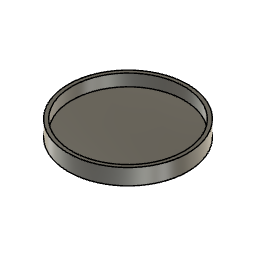
Piston Hood 1 (Autodesk Fusion 360 design; units mm, degrees)
Autodesk Fusion 360 part; units mm, degrees
sketch "Sketch1" plane through (0, 0, 0) normal (0, 0, 1) x (1, 0, 0) in component "Component"
  line L0 (3.8891, 2.4749) -> (5.2486, 3.8344)
  circle A0 centre (0, 0) radius 6.5
  line L1 (-2.4749, 3.8891) -> (-3.8344, 5.2486)
  circle A1 centre (0, 0) radius 7.05
  line L2 (3.182, 3.182) -> (2.4749, 3.8891)
  line L3 (-3.182, 3.182) -> (-3.8891, 2.4749)
  line L4 (-3.182, -3.182) -> (-2.4749, -3.8891)
  line L5 (-3.8891, -2.4749) -> (-5.2486, -3.8344)
  line L6 (2.4749, -3.8891) -> (3.8344, -5.2486)
  line L7 (-2.4749, -3.8891) -> (-3.8344, -5.2486)
  line L8 (3.182, -3.182) -> (2.4749, -3.8891)
  line L9 (-3.182, -3.182) -> (-3.8891, -2.4749)
  circle A2 centre (0, 0) radius 7.5
  line L10 (3.182, 3.182) -> (3.8891, 2.4749)
  line L11 (-3.8891, 2.4749) -> (-5.2486, 3.8344)
  line L12 (-3.182, 3.182) -> (-2.4749, 3.8891)
  line L13 (3.8891, -2.4749) -> (5.2486, -3.8344)
  line L14 (3.182, -3.182) -> (3.8891, -2.4749)
  line L15 (2.4749, 3.8891) -> (3.8344, 5.2486)
  circle A3 centre (0, 0) radius 1.5
  dimension "d1" = 15
  dimension "d2" = 14.1
  dimension "d3" = 13
  dimension "d8" = 3
  constraint coincident A0.centre A1.centre
  constraint concentric A1 A2
  constraint concentric A0 A3
  measures "d1" diameter of A2
  measures "d2" diameter of A1
  measures "d3" diameter of A0
  measures "d8" diameter of A3
extrude "Extrude1" add sketch "Sketch1" along normal blind 2 contours A2 in component "Component"
extrude "Extrude2" add sketch "Sketch1" along normal blind 0.5 contours L0 A0 L2 L10 L15 | L0 A0 L1 L2 L3 L4 L5 L6 L7 L8 L9 L10 L11 L12 L13 L14 L15 | A0 L6 L8 L13 L14 | A0 L1 L3 L11 L12 | A0 L4 L5 L7 L9 | A1 | A3 in component "Component"
extrude "Extrude3" add sketch "Sketch1" along normal blind 30.5 contours A3 in component "Component"
extrude "Extrude4" cut 1 faces at (0.567, -0.5383, 30.5) along direction (0, 0, -1) blind 30 in component "Component"
extrude "Extrude5" add sketch "Sketch1" along normal blind 30.5 contours A3 in component "Component"
extrude "Extrude6" cut 1 faces at (0.567, -0.5383, 30.5) along direction (0, 0, -1) blind 30 in component "Component"
component "Component" placed x (1, 0, 0) y (0, 1, 0) z (0, 0, 1) at (0, 0, 0)
